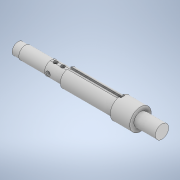
# Autodesk Inventor part: eixo 2
Saved by Autodesk Inventor 2022.1 (Build 261234020, 234B)
## iProperties
Created: 2023-09-01
Part Number: eixo 2
Material: Generic
Document SubType Name: Modeling
Designer: SENAI
Density: 1 g/cm^3
Appearance: Default
Author: SENAI
Autodesk Inventor part; units mm, degrees
sketch "Sketch1" plane through (0, 0, 0) normal (0, 0, 1) x (1, 0, 0)
  line L0 (0, 0) -> (302, 0)
  line L1 (0, 0) -> (0, 12.5)
  line L2 (0, 12.5) -> (15, 12.5)
  line L3 (15, 12.5) -> (15, 13.5)
  line L4 (15, 13.5) -> (70, 13.5)
  line L5 (70, 13.5) -> (70, 14.5)
  line L6 (70, 14.5) -> (107, 14.5)
  line L7 (107, 14.5) -> (107, 18.5)
  line L8 (107, 18.5) -> (216, 18.5)
  line L9 (216, 18.5) -> (216, 22.5)
  line L10 (302, 0) -> (302, 14)
  line L11 (302, 14) -> (257, 14)
  line L12 (216, 22.5) -> (257, 22.5)
  line L13 (257, 22.5) -> (257, 14)
  dimension "d0" = 302
  dimension "d1" = 12.5
  dimension "d2" = 15
  dimension "d3" = 1
  dimension "d4" = 55
  dimension "d5" = 1
  dimension "d6" = 37
  dimension "d7" = 4
  dimension "d8" = 109
  dimension "d9" = 4
  dimension "d10" = 14
  dimension "d11" = 45
  constraints: 28 end point, 10 perpendicular, 2 horizontal, 2 vertical
  measures "d0" distance of L0.start L0.end
  measures "d1" distance of L0.start L1.end
  measures "d2" distance of L1.end L2.end
  measures "d3" distance of L2.end L3.end
  measures "d4" distance of L3.end L4.end
  measures "d5" distance of L4.end L5.end
  measures "d6" distance of L5.end L6.end
  measures "d7" distance of L6.end L7.end
  measures "d8" distance of L7.end L8.end
  measures "d9" distance of L8.end L9.end
  measures "d10" distance of L0.end L10.end
  measures "d11" distance of L10.end L11.end
revolve "Revolution1" add sketch "Sketch1" angle 360 about axis through (0, 0, 0) along (1, 0, 0)
ref_plane "Work Plane1" through (0, 17.5, 0) normal (0, 1, 0) x (-1, 0, 0)
ref_plane "Work Plane2" through (0, 14.25, 0) normal (0, 1, 0) x (-1, 0, 0)
sketch "Sketch3" plane through (0, 14.25, 0) normal (0, 1, 0) x (-1, 0, 0)
  line L0 (-70, -4) -> (-220, -4)
  line L1 (-220, -4) -> (-220, 4)
  line L2 (-216, 22.5) -> (-216, -22.5) projected
  line L3 (-220, 4) -> (-70, 4)
  line L4 (-70, -4) -> (-70, 4)
  line L5 (-70, 14.5) -> (-70, -14.5) projected
  point P0 (0, 0)
  dimension "d17" = 150
  dimension "d18" = 8
  dimension "d19" = 150
  constraints: 8 end point, 1 collinear, 1 horizontal, 1 perpendicular
  measures "d17" distance of L0.start L0.end
  measures "d18" distance of L0.end L1.end
  measures "d19" distance of L1.end L3.end
extrude "Extrusion1" cut sketch "Sketch3" along normal blind 10
fillet "Fillet1" radius 10 1 edges at (220, 14.25, 0)
sketch "Sketch4" plane through (0, 14.25, 0) normal (0, 1, 0) x (1, 0, 0)
  circle A0 centre (79, 0) radius 4
  circle A1 centre (94, 0) radius 4
  line L0 (70, -2.681) -> (70, 2.681) projected
  point P0 (0, 0)
  dimension "d23" = 8
  dimension "d24" = 8
  constraints: 2 centre point
  measures "d23" diameter of A0
  measures "d24" diameter of A1
extrude "Extrusion2" cut sketch "Sketch4" against normal blind 9
ref_plane "Work Plane3" through (0, 0, -14.5) normal (0, 0, 1) x (1, 0, 0)
sketch "Sketch5" plane through (0, 0, -14.5) normal (0, 0, 1) x (1, 0, 0)
  circle A0 centre (77.4995, -0.0611) radius 4.5
  line L0 (70, -14.5) -> (70, 14.25) projected
  point P0 (0, 0)
  dimension "d31" = 9
  constraints: 1 centre point
  measures "d31" diameter of A0
extrude "Extrusion3" cut sketch "Sketch5" along normal blind 30
body "Solid1"
